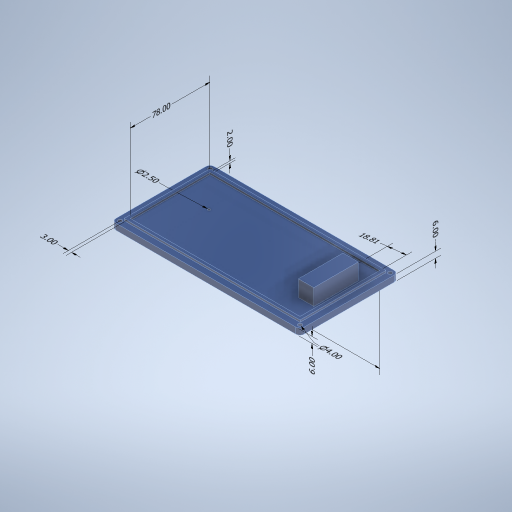
# Autodesk Inventor part: Tapa principal
Saved by Autodesk Inventor 2023 (Build 270158000, 158)
## iProperties
Created: 2023-03-20
Part Number: Tapa principal
Material: Plástico PET
Document SubType Name: Modeling
Designer: sergi
Density: 1.541 g/cm^3
Appearance: Satinado con motas - Azul
Author: sergi
Autodesk Inventor part; units mm, degrees
ref_plane "YZ Plane" through (0, 0, 0) normal (1, 0, 0) x (0, 1, 0)
ref_plane "XZ Plane" through (0, 0, 0) normal (0, 1, 0) x (-1, 0, 0)
ref_plane "XY Plane" through (0, 0, 0) normal (0, 0, 1) x (1, 0, 0)
sketch "Boceto1" plane through (0, 0, 0) normal (0, 1, 0) x (-1, 0, 0)
  line L0 (-44, 24) -> (44, 24)
  line L1 (46, 22) -> (46, -22)
  line L2 (44, -24) -> (-44, -24)
  line L3 (-46, -22) -> (-46, 22)
  line L4 (-46, 24) -> (46, -24) construction
  line L5 (46, 24) -> (-46, -24) construction
  arc A0 (44, -24) -> (46, -22) centre (44, -22) ccw
  arc A1 (-46, -22) -> (-44, -24) centre (-44, -22) ccw
  arc A2 (-44, 24) -> (-46, 22) centre (-44, 22) ccw
  arc A3 (46, 22) -> (44, 24) centre (44, 22) ccw
  point P0 (0, 0)
  dimension "d0" = 92
  dimension "d1" = 48
  dimension "d2" = 2
  constraints: 12 end point, 8 point on circle, 8 point on line, 8 tangent, 4 centre point, 3 equal radius, 2 midpoint, 2 parallel, 1 horizontal, 1 perpendicular
  measures "d0" distance of L4.end L5.end
  measures "d1" distance of L5.start L4.end
  measures "d2" radius of A0
extrude "Extrusión1" add sketch "Boceto1" along normal blind 3
sketch "Boceto2" plane through (0, 3, 0) normal (0, 1, 0) x (1, 0, 0)
  line L0 (43, -21) -> (-43, -21)
  line L1 (-43, -21) -> (-43, 21)
  line L2 (-43, 21) -> (43, 21)
  line L3 (43, 21) -> (43, -21)
  line L4 (43, -21) -> (-43, 21) construction
  line L5 (-43, -21) -> (43, 21) construction
  line L6 (44, 24) -> (-44, 24) projected
  line L7 (46, -22) -> (46, 22) projected
  line L8 (41.5, -19.5) -> (-41.5, -19.5)
  line L9 (-41.5, -19.5) -> (-41.5, 19.5)
  line L10 (-41.5, 19.5) -> (41.5, 19.5)
  line L11 (41.5, 19.5) -> (41.5, -19.5)
  line L12 (41.5, -19.5) -> (-41.5, 19.5) construction
  line L13 (-41.5, -19.5) -> (41.5, 19.5) construction
  point P0 (0, 0)
  dimension "d5" = 3
  dimension "d6" = 3
  dimension "d7" = 1.5
  dimension "d8" = 1.5
  constraints: 24 end point, 4 midpoint, 4 parallel, 2 horizontal, 2 perpendicular
  measures "d5" distance between parallel lines of L6 L2
  measures "d6" distance between parallel lines of L7 L3
  measures "d7" distance between parallel lines of L3 L11
  measures "d8" distance between parallel lines of L2 L10
extrude "Extrusión2" add sketch "Boceto2" along normal blind 1
sketch "Sketch7" plane through (0, 3, 0) normal (0, 1, 0) x (1, 0, 0)
  arc A0 (46, 22) -> (44, 24) centre (44, 22) ccw projected
  circle A1 centre (44, 22) radius 1
  arc A2 (44, -24) -> (46, -22) centre (44, -22) ccw projected
  circle A3 centre (44, -22) radius 1
  arc A4 (-46, -22) -> (-44, -24) centre (-44, -22) ccw projected
  circle A5 centre (-44, -22) radius 1
  arc A6 (-44, 24) -> (-46, 22) centre (-44, 22) ccw projected
  circle A7 centre (-44, 22) radius 1
  point P0 (0, 0)
  dimension "d46" = 2
  dimension "d47" = 2
  dimension "d48" = 2
  dimension "d49" = 2
  constraints: 4 centre point, 4 coincident
  measures "d46" diameter of A1
  measures "d47" diameter of A3
  measures "d48" diameter of A5
  measures "d49" diameter of A7
extrude "Extrusion3" cut sketch "Sketch7" against normal blind 3
sketch "Boceto8" plane through (0, 3, 0) normal (0, 1, 0) x (1, 0, 0)
  line L0 (32.15, 7.35) -> (36.5, 7.35)
  line L1 (36.5, 7.35) -> (36.5, -7.4)
  line L2 (36.5, -7.4) -> (32.15, -7.4)
  line L3 (32.15, -7.4) -> (32.15, 7.35)
  line L4 (41.5, 19.5) -> (41.5, -19.5) projected
  line L5 (-41.5, 19.5) -> (41.5, 19.5) projected
  point P0 (0, 0)
  dimension "d58" = 14.75
  dimension "d59" = 4.35
  dimension "d60" = 5
  dimension "d61" = 12.15
  constraints: 8 end point, 2 parallel, 1 horizontal, 1 perpendicular
  measures "d58" distance of L2.end L0.start
  measures "d59" distance of L0.start L0.end
  measures "d60" distance between parallel lines of L4 L1
  measures "d61" distance between parallel lines of L5 L0
extrude "Extrusión4" cut sketch "Boceto8" against normal blind 10
sketch "Boceto9" plane through (0, 0, 0) normal (0, -1, 0) x (1, 0, 0)
  line L0 (36.5, -7.35) -> (36.5, 7.4) projected
  line L1 (32.15, 7.4) -> (32.15, -7.35) projected
  line L2 (36.5, -7.35) -> (32.15, -7.35)
  line L3 (32.15, -7.35) -> (32.15, 7.4)
  line L4 (32.15, 7.4) -> (36.5, 7.4)
  line L5 (36.5, 7.4) -> (36.5, -7.35)
  line L6 (38.5, -9.35) -> (30.15, -9.35)
  line L7 (30.15, -9.35) -> (30.15, 9.4)
  line L8 (30.15, 9.4) -> (38.5, 9.4)
  line L9 (38.5, 9.4) -> (38.5, -9.35)
  point P0 (0, 0)
  point P1 (32.15, -7.35)
  point P2 (36.5, 7.4)
  dimension "d67" = 2
  dimension "d68" = 2
  dimension "d69" = 2
  dimension "d70" = 2
  constraints: 16 end point, 4 parallel, 2 horizontal, 2 perpendicular
  measures "d67" distance between parallel lines of L7 L1
  measures "d68" distance between parallel lines of L8 L4
  measures "d69" distance between parallel lines of L9 L0
  measures "d70" distance between parallel lines of L6 L2
extrude "Extrusión5" cut sketch "Boceto9" against normal blind 1
sketch "Boceto11" plane through (0, 3, 0) normal (0, 1, 0) x (1, 0, 0)
  line L0 (38.65, 9.85) -> (32.15, 9.85)
  line L1 (32.15, 9.85) -> (32.15, -9.9)
  line L2 (32.15, -9.9) -> (38.65, -9.9)
  line L3 (38.65, -9.9) -> (38.65, 9.85)
  line L4 (41.5, 19.5) -> (41.5, -19.5) projected
  line L5 (32.15, -7.4) -> (32.15, 7.35) projected
  line L6 (36.5, -7.4) -> (32.15, -7.4) projected
  line L7 (32.15, 7.35) -> (36.5, 7.35) projected
  line L8 (39.65, 10.85) -> (32.15, 10.85)
  line L9 (32.15, 10.85) -> (32.15, -10.9)
  line L10 (32.15, -10.9) -> (39.65, -10.9)
  line L11 (39.65, -10.9) -> (39.65, 10.85)
  point P0 (0, 0)
  dimension "d75" = 6.5
  dimension "d76" = 9.35
  dimension "d77" = 2.85
  dimension "d78" = 2.5
  dimension "d79" = 2.5
  dimension "d80" = 1
  dimension "d81" = 1
  dimension "d82" = 1
  constraints: 16 end point, 4 parallel, 2 horizontal, 2 perpendicular
  measures "d75" distance of L1.end L2.end
  measures "d76" distance between parallel lines of L4 L5
  measures "d77" distance between parallel lines of L4 L3
  measures "d78" distance between parallel lines of L2 L6
  measures "d79" distance between parallel lines of L0 L7
  measures "d80" distance between parallel lines of L8 L0
  measures "d81" distance between parallel lines of L10 L2
  measures "d82" distance between parallel lines of L11 L3
extrude "Extrusión6" add sketch "Boceto11" along normal blind 7 contours L0 L9 L8 L11 L10 L2 L3
sketch "Boceto12" plane through (0, 10, 0) normal (0, 1, 0) x (1, 0, 0)
  line L0 (32.15, 10.85) -> (39.65, 10.85) projected
  line L1 (32.15, -10.9) -> (32.15, -9.9) projected
  line L2 (39.65, 10.85) -> (32.15, 10.85)
  line L3 (32.15, 10.85) -> (32.15, -10.9)
  line L4 (32.15, -10.9) -> (39.65, -10.9)
  line L5 (39.65, -10.9) -> (39.65, 10.85)
  point P0 (0, 0)
  constraints: 8 end point, 2 parallel, 1 horizontal, 1 perpendicular
extrude "Extrusión7" add sketch "Boceto12" along normal blind 1
sketch "Boceto13" plane through (0, 3, 0) normal (0, 1, 0) x (1, 0, 0)
  line L0 (-41.5, 19.5) -> (-41.5, -19.5) projected
  line L1 (-41.5, -19.5) -> (-27, -19.5)
  line L2 (-41.5, -19.5) -> (41.5, -19.5) projected
  line L3 (-27, -19.5) -> (-27, 4.5)
  circle A0 centre (-27, 4.5) radius 0.625
  point P0 (0, 0)
  dimension "d93" = 14.5
  dimension "d94" = 24
  dimension "d95" = 1.25
  constraints: 4 end point, 1 centre point, 1 coincident, 1 perpendicular, 1 point on line
  measures "d93" distance of L0.end L1.end
  measures "d94" distance of L1.end L3.end
  measures "d95" diameter of A0
extrude "Extrusión8" cut sketch "Boceto13" against normal blind 3
scale "Escala1" factors (2, 2, 2) then translate (0, 0, 0) bodies 1
